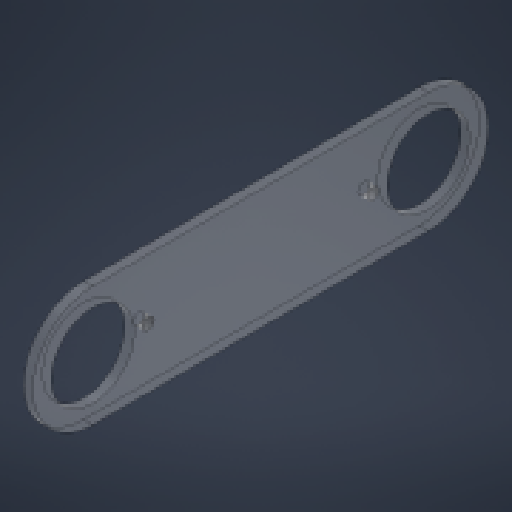
# Autodesk Inventor part: PLATE,KICKER,MOTOR,SUPPORT
Saved by Autodesk Inventor 2026.1 (Build 301233020, 233B)
## iProperties
Created: 2026-02-14
Part Number: PLATE,KICKER,MOTOR,SUPPORT
Material: Polycarbonate, Clear
Document SubType Name: Sheet Metal
Designer: Owen L
Mass: 18.2822 g
Surface Area: 113.913 cm^2
Volume: 15.2352 cm^3
Density: 1.2 g/cm^3
Sheet Metal Rule: Default
Appearance: Polycarbonate - Clear
Author: Owen L
Autodesk Inventor part; units mm, degrees
ref_plane "YZ Plane" through (0, 0, 0) normal (1, 0, 0) x (0, 1, 0)
ref_plane "XZ Plane" through (0, 0, 0) normal (0, 1, 0) x (-1, 0, 0)
ref_plane "XY Plane" through (0, 0, 0) normal (0, 0, 1) x (1, 0, 0)
sketch "Sketch1" plane through (0, 0, 0) normal (1, 0, 0) x (0, 1, 0)
  arc A0 (-20.6375, 0) -> (20.6375, 0) centre (0, 0) ccw
  arc A1 (20.6375, 115.5112) -> (-20.6375, 115.5112) centre (0, 115.5112) ccw
  line L0 (-20.6375, 115.5112) -> (-20.6375, 0)
  line L1 (20.6375, 0) -> (20.6375, 115.5112)
  dimension "d0" = 115.5112
  dimension "d1" = 41.275
  measures "d0" distance of point (0, 0) A1.centre
  measures "d1" distance between parallel lines of L1 L0
extrude "Plate1" add sketch "Sketch1" along normal blind 3.175
sketch "Sketch2" plane through (3.175, 0, 0) normal (1, 0, 0) x (0, 0, -1)
  point P0 (0, 0)
  point P1 (0, 0)
  point P2 (0, 0)
  point P3 (-115.5112, 0)
  dimension "d21" = 115.5112
  constraints: 1 coincident, 1 horizontal alignment
  measures "d21" distance of point (-115.511, 0) point (0, 0)
hole "Hole1" at (3.175, 0, 0) at (3.175, 0, 115.5112) direction (-1, 0, 0) diameter 28.575 depth 3.175 tip angle 118
sketch "Sketch3" plane through (3.175, 0, 0) normal (1, 0, 0) x (0, 0, -1)
  circle A0 centre (0, 0) radius 15.5575 construction
  point P0 (-18.288, 0)
  point P1 (-115.5112, 0)
  point P2 (-97.2232, 0)
  dimension "d10" = 31.115
  dimension "d13" = 18.288
  dimension "d22" = 115.5112
  dimension "d23" = 18.288
  constraints: 3 horizontal alignment, 1 centre point, 1 coincident
  measures "d10" diameter of A0
  measures "d13" distance of point (-18.288, 0) point (0, 0)
  measures "d22" distance of point (0, 0) point (-115.511, 0)
  measures "d23" distance of point (-115.511, 0) point (-97.223, 0)
hole "Hole2" at (3.175, 0, 18.288) at (3.175, 0, 97.2232) direction (-1, 0, 0) diameter 3.9624 depth 13.6144 tip angle 118 thread size "10-32 UNF" class "2B" standard "ANSI Unified Screw Threads"
equation "\"d21\" = d0"
equation "\"d8\" = Thickness"
equation "\"d2\" = Thickness"
equation "\"d22\" = d0"
equation "\"d23\" = d13"
equation "\"BendRadius\" = Thickness"
equation "\"BendReliefWidth\" = Thickness"
equation "\"BendReliefDepth\" = 0.5 * Thickness"
equation "\"CornerReliefSize\" = 4 * Thickness"
equation "\"MinimumRemnant\" = 2 * Thickness"
equation "\"TransitionRadius\" = BendRadius"
equation "\"JacobiRadiusSize\" = BendRadius"
equation "\"GapSize\" = Thickness"
equation "\"Thickness\" = 3.175"
body "Solid1"
